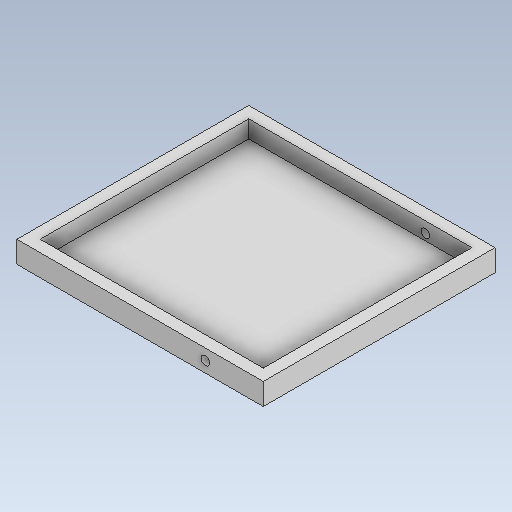
# Autodesk Inventor part: baseplate
Saved by Autodesk Inventor 2020.1 (Build 241239000, 239)
## iProperties
Created: 2019-09-10
Part Number: baseplate
Material: Generic
Document SubType Name: Modeling
Designer: Julian
Density: 1 g/cm^3
Appearance: Default
Author: Julian
Autodesk Inventor part; units mm, degrees
ref_plane "YZ Plane" through (0, 0, 0) normal (1, 0, 0) x (0, 1, 0)
ref_plane "XZ Plane" through (0, 0, 0) normal (0, 1, 0) x (-1, 0, 0)
ref_plane "XY Plane" through (0, 0, 0) normal (0, 0, 1) x (1, 0, 0)
sketch "Sketch2" plane through (0, 0, 0) normal (0, 1, 0) x (-1, 0, 0)
  line L0 (0, 0) -> (-170, 0)
  line L1 (-170, 0) -> (-170, -160)
  line L2 (-170, -160) -> (0, -160)
  line L3 (0, -160) -> (0, 0)
  line L4 (-8, -8) -> (-162, -8)
  line L5 (-162, -8) -> (-162, -152)
  line L6 (-162, -152) -> (-8, -152)
  line L7 (-8, -152) -> (-8, -8)
  dimension "d0" = 170
  dimension "d1" = 160
  dimension "d2" = 154
  dimension "d3" = 144
  dimension "d4" = 8
  dimension "d5" = 8
  constraints: 16 end point, 4 parallel, 2 horizontal, 2 perpendicular
  measures "d0" distance of L2.end L1.end
  measures "d1" distance of L1.end L0.end
  measures "d2" distance of L6.end L5.end
  measures "d3" distance of L5.end L4.end
  measures "d4" distance between parallel lines of L4 L0
  measures "d5" distance between parallel lines of L7 L3
extrude "Extrusion1" add sketch "Sketch2" along normal blind 15
extrude "Extrusion2" add sketch "Sketch2" along normal blind 3 contours L7 L6 L5 L4
sketch "Sketch3" plane through (0, 0, 0) normal (0, 0, 1) x (1, 0, 0)
  line L0 (0, 0) -> (0, 7.5)
  line L1 (0, 0) -> (0, 15) projected
  line L2 (0, 7.5) -> (170, 7.5)
  line L3 (170, 0) -> (170, 15) projected
  line L4 (0, 7.5) -> (40, 7.5)
  line L5 (170, 7.5) -> (130, 7.5)
  dimension "d10" = 40
  dimension "d11" = 40
  constraints: 8 end point, 2 midpoint, 2 point on line
  measures "d10" distance of L0.end L4.end
  measures "d11" distance of L2.end L5.end
hole "Hole1" at (130, 7.5, 0) direction (0, 0, -1) diameter 6 depth 160
body "Solid1"
